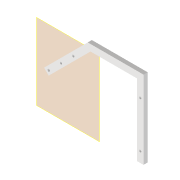
# Autodesk Inventor part: NematostellaImager_illuminationmount
Saved by Autodesk Inventor 2022.5 (Build 265521000, 521)
## iProperties
Created: 2023-11-06
Part Number: NematostellaImager_illuminationmount
Material: Generisch
Document SubType Name: Modeling
Designer: diederichbenedict
Density: 1 g/cm^3
Appearance: Vorgabe
Author: diederichbenedict
Autodesk Inventor part; units mm, degrees
ref_plane "YZ Plane" through (0, 0, 0) normal (1, 0, 0) x (0, 1, 0)
ref_plane "XZ Plane" through (0, 0, 0) normal (0, 1, 0) x (-1, 0, 0)
ref_plane "XY Plane" through (0, 0, 0) normal (0, 0, 1) x (1, 0, 0)
ref_plane "Arbeitsebene1" through (0, 0, 0) normal (0, 0, 1) x (1, 0, 0)
sketch "Skizze1" plane through (0, 0, 0) normal (0, 0, 1) x (1, 0, 0)
  circle A0 centre (41.3693, 78.2732) radius 1.4 projected
  circle A1 centre (11.3693, 48.2732) radius 1.49 projected
  line L0 (5.7124, 48.2732) -> (41.3693, 83.9301) projected
  line L1 (47.0261, 78.2732) -> (11.3693, 42.6164) projected
  line L2 (41.3693, 83.9301) -> (47.0261, 78.2732) projected
  line L3 (11.3693, 42.6164) -> (5.7124, 48.2732) projected
  line L4 (47.0261, 78.2732) -> (41.3693, 83.9301)
  line L5 (41.3693, 83.9301) -> (59.0469, 101.6077)
  line L6 (59.0469, 101.6077) -> (64.7038, 95.9509)
  line L7 (64.7038, 95.9509) -> (47.0261, 78.2732)
  line L8 (59.0469, 101.6077) -> (59.0469, 93.6077)
  line L9 (59.0469, 93.6077) -> (119.0469, 93.6077)
  line L10 (119.0469, 93.6077) -> (119.0469, 101.6077)
  line L11 (119.0469, 101.6077) -> (59.0469, 101.6077)
  line L12 (119.0469, 101.6077) -> (119.0469, 6.2524)
  line L13 (119.0469, 6.2524) -> (127.0469, 6.2524)
  line L14 (127.0469, 6.2524) -> (127.0469, 101.6077)
  line L15 (127.0469, 101.6077) -> (119.0469, 101.6077)
  circle A2 centre (26.3693, 63.2732) radius 1.4
  point P0 (0, 0)
  point P1 (62.3606, 93.6077)
  dimension "d0" = 25
  dimension "d1" = 8
  dimension "d2" = 60
  dimension "d3" = 8
  dimension "d10" = 2.8
  constraints: 24 end point, 6 parallel, 3 perpendicular, 2 point on line, 1 centre point, 1 vertical
  measures "d0" distance of L0.end L5.end
  measures "d1" distance of L5.end L8.end
  measures "d2" distance of L9.end L8.end
  measures "d3" distance of L13.end L12.end
  measures "d10" diameter of A2
extrude "Extrusion1" add sketch "Skizze1" along normal blind 5
sketch "Skizze2" plane through (0, 0, 5) normal (0, 0, 1) x (1, 0, 0)
  line L0 (127.0469, 6.2524) -> (127.0469, 101.6077) projected
  line L1 (127.0469, 101.6077) -> (59.0469, 101.6077) projected
  line L2 (59.0469, 101.6077) -> (5.7124, 48.2732) projected
  line L3 (5.7124, 48.2732) -> (11.3693, 42.6164) projected
  line L4 (11.3693, 42.6164) -> (62.3606, 93.6077) projected
  line L5 (62.3606, 93.6077) -> (119.0469, 93.6077) projected
  line L6 (119.0469, 93.6077) -> (119.0469, 6.2524) projected
  line L7 (119.0469, 6.2524) -> (127.0469, 6.2524) projected
  circle A0 centre (11.3693, 48.2732) radius 1.49 projected
  circle A1 centre (41.3693, 78.2732) radius 1.4 projected
  circle A2 centre (123.0469, 18.77) radius 1.4
  circle A3 centre (123.0469, 74.9405) radius 1.4
  point P0 (0, 0)
  dimension "d6" = 2.8
  dimension "d7" = 2.8
  constraints: 2 centre point
  measures "d6" diameter of A2
  measures "d7" diameter of A3
extrude "Extrusion2" cut sketch "Skizze2" against normal blind 5 contours A2 | A3
